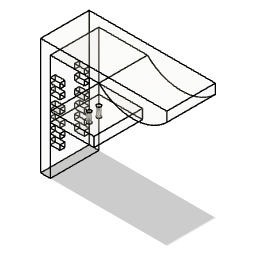
clamp v5 (Autodesk Fusion 360 design; units mm, degrees)
Autodesk Fusion 360 part; units mm, degrees
sketch "草图1" plane through (0, 0, 0) normal (0, 1, 0) x (1, 0, 0) in component "Component"
  line L0 (-30, 25) -> (30, 25)
  line L1 (30, 25) -> (30, -25)
  line L2 (30, -25) -> (-30, -25)
  line L3 (-30, -25) -> (-30, 25)
  line L4 (-30, 25) -> (30, -25) construction
  line L5 (30, 25) -> (-30, -25) construction
  dimension "d1" = 60
  dimension "d2" = 50
  constraint horizontal L0
  constraint perpendicular L0 L1
  constraint parallel L0 L2
  constraint parallel L1 L3
  constraint coincident L4 origin
  constraint coincident L5 origin
  measures "d1" distance of L0.start L0.end
  measures "d2" distance of L0.start L2.end
extrude "拉伸1" add sketch "草图1" along normal blind 10 makes body 1 in component "Component"
sketch "草图2" plane through (0, 10, 0) normal (0, 1, 0) x (-1, 0, 0) in component "Component"
  line L0 (30, 25) -> (-30, 25)
  line L1 (-30, 25) -> (-30, -25)
  line L2 (-30, -25) -> (30, -25)
  line L3 (30, -25) -> (30, 25)
  line L4 (30, -25) -> (20, -25)
  line L5 (20, -25) -> (20, 25)
  line L6 (20, 25) -> (30, 25)
  line L7 (30, 25) -> (30, -25)
  dimension "d5" = 10
  constraint horizontal L4
  constraint vertical L5
  constraint horizontal L6
  constraint vertical L7
  constraint coincident L0 L5.end
  constraint coincident L2.end L3.start
  measures "d5" distance of L2.end L4.end
extrude "拉伸2" add sketch "草图2" along normal blind 60 contours L0 L2 L3 L4 L5 L6 L7 bodies 1 in component "Component"
sketch "草图3" plane through (-20, 0, 0) normal (1, 0, 0) x (0, 0, -1) in component "Component"
  line L0 (-25, 10) -> (25, 10)
  line L1 (25, 10) -> (25, 70)
  line L2 (25, 70) -> (-25, 70)
  line L3 (-25, 70) -> (-25, 10)
  line L4 (-25, 70) -> (25, 70)
  line L5 (25, 70) -> (25, 60)
  line L6 (25, 60) -> (-25, 60)
  line L7 (-25, 60) -> (-25, 70)
  dimension "d8" = 10
  constraint horizontal L4
  constraint vertical L5
  constraint horizontal L6
  constraint vertical L7
  constraint coincident L1 L5.end
  constraint coincident L2.end L3.start
  measures "d8" distance of L2.end L6.end
extrude "拉伸3" add sketch "草图3" along normal blind 120 contours L1 L2 L3 L4 L5 L6 L7 bodies 1 in component "Component"
sketch "草图1 (2)" plane through (0, 0, 25) normal (0, 0, 1) x (1, 0, 0)
  line L0 (-30, 0) -> (30, 0)
  line L1 (30, 0) -> (30, 10)
  line L2 (30, 10) -> (-20, 10)
  line L3 (-20, 10) -> (-20, 60)
  line L4 (-20, 60) -> (100, 60)
  line L5 (100, 60) -> (100, 70)
  line L6 (100, 70) -> (-30, 70)
  line L7 (-30, 70) -> (-30, 0)
  arc A0 (30, 60) -> (100, 60) centre (65, 95.7071) ccw
  dimension "d14" = 50
  dimension "d15" = 50
  constraint coincident L4.end L5.start
  constraint coincident L4 A0.start
  measures "d14" radius of A0
  measures "d15" distance of L3.end A0.start
extrude "拉伸4" add sketch "草图1 (2)" against normal blind 50 contours L4 A0 bodies 1 in component "Component"
sketch "草图2 (2)" plane through (0, 0, 0) normal (0, -1, 0) x (1, 0, 0)
  line L0 (30, 25) -> (-30, 25)
  line L1 (-30, 25) -> (-30, -25)
  line L2 (-30, -25) -> (30, -25)
  line L3 (30, -25) -> (30, 25)
  line L4 (-20, -25) -> (-20, 25)
  line L5 (-30, 25) -> (-20, 25)
  line L6 (-20, 25) -> (-20, -25)
  line L7 (-20, -25) -> (-30, -25)
  line L8 (-30, -25) -> (-30, 25)
  constraint horizontal L5
  constraint vertical L6
  constraint horizontal L7
  constraint vertical L8
  constraint coincident L4.start L6.end
  constraint coincident L0.end L1.start
extrude "拉伸5" add sketch "草图2 (2)" along normal blind 50 contours L0 L1 L2 L4 L5 L6 L7 L8 bodies 1 in component "Component"
sketch "草图3 (2)" plane through (0, 0, 0) normal (0, -1, 0) x (1, 0, 0)
  line L0 (-20, 25) -> (-20, -25)
  line L1 (-20, -25) -> (30, -25)
  line L2 (30, -25) -> (30, 25)
  line L3 (30, 25) -> (-20, 25)
  dimension "d21" = 20
  measures "d21" distance of origin L0
ref_plane "工作平面2" through (-20, 0, 0) normal (1, 0, 0) x (0, 1, 0)
split "分割1" by plane through (-20, 0, 0) normal (1, 0, 0) bodies 1 makes body 2 at (20, 70, -8.3333) makes body 3 at (-3.3333, 0, -8.3333) in component "Component"
combine "合并1" operation add target body 2 tool bodies 1 in component "Component"
sketch "草图4" plane through (-20, 0, 0) normal (-1, 0, 0) x (0, 0, 1)
  line L0 (25, 10) -> (-25, 10)
  line L1 (-25, 10) -> (-25, 0)
  line L2 (-25, 0) -> (25, 0)
  line L3 (25, 0) -> (25, 10)
  line L4 (-15, 7) -> (-10, 7)
  line L5 (-10, 7) -> (-10, 2)
  line L6 (-10, 2) -> (-15, 2)
  line L7 (-15, 2) -> (-15, 7)
  line L8 (10, 7) -> (15, 7)
  line L9 (15, 7) -> (15, 2)
  line L10 (15, 2) -> (10, 2)
  line L11 (10, 2) -> (10, 7)
  dimension "d24" = 5
  dimension "d25" = 5
  dimension "d26" = 5
  dimension "d27" = 10
  dimension "d28" = 3
  dimension "d29" = 5
  dimension "d30" = 5
  dimension "d31" = 10
  dimension "d32" = 3
  constraint horizontal L4
  constraint vertical L5
  constraint horizontal L6
  constraint vertical L7
  constraint horizontal L8
  constraint vertical L9
  constraint horizontal L10
  constraint vertical L11
  measures "d24" distance of L4.start L4.end
  measures "d25" distance of L4.start L6.end
  measures "d26" distance of L4.start L4.end
  measures "d27" distance of origin L5
  measures "d28" distance of L0 L4
  measures "d29" distance of L8.start L8.end
  measures "d30" distance of L8.start L10.end
  measures "d31" distance of L11 origin
  measures "d32" distance of L0 L8
extrude "拉伸6" add sketch "草图4" along normal blind 8 contours L4 L5 L6 L7 | L8 L9 L10 L11 bodies 3 in component "Component"
sketch "草图5" plane through (-20, 0, 0) normal (1, 0, 0) x (0, 0, -1)
  line L0 (25, 60) -> (-25, 60)
  line L1 (-25, 60) -> (-25, -50)
  line L2 (-25, -50) -> (25, -50)
  line L3 (25, -50) -> (25, 60)
  line L4 (-10, 2) -> (-15, 2)
  line L5 (-15, 2) -> (-15, 7)
  line L6 (-15, 7) -> (-10, 7)
  line L7 (-10, 7) -> (-10, 2)
  line L8 (15, 2) -> (10, 2)
  line L9 (10, 2) -> (10, 7)
  line L10 (10, 7) -> (15, 7)
  line L11 (15, 7) -> (15, 2)
  line L12 (-15, 7) -> (-10, 7)
  line L13 (-10, 7) -> (-10, 2)
  line L14 (-10, 2) -> (-15, 2)
  line L15 (-15, 2) -> (-15, 7)
  line L16 (10, 7) -> (15, 7)
  line L17 (15, 7) -> (15, 2)
  line L18 (15, 2) -> (10, 2)
  line L19 (10, 2) -> (10, 7)
  constraint horizontal L12
  constraint vertical L13
  constraint horizontal L14
  constraint vertical L15
  constraint coincident L4.start L7.end
  constraint coincident L5.end L6.start
  constraint horizontal L16
  constraint vertical L17
  constraint horizontal L18
  constraint vertical L19
  constraint coincident L8.start L11.end
  constraint coincident L9.end L10.start
extrude "拉伸7" cut sketch "草图5" against normal blind 10 contours L4 L5 L6 L7 L12 L13 L14 L15 | L8 L9 L10 L11 L16 L17 L18 L19 bodies 2 in component "Component"
extrude "拉伸8" add 2 faces at (-28, 5.3333, 11.6667) (-28, 5.3333, -13.3333) along direction (-1, 0, 0) blind 2 on bodies 3 bodies 3 in component "Component"
sketch "草图6" plane through (-30, 0, 0) normal (-1, 0, 0) x (0, 0, 1)
  line L0 (10, 2) -> (10, 7)
  line L1 (10, 7) -> (15, 7)
  line L2 (15, 7) -> (15, 2)
  line L3 (15, 2) -> (10, 2)
  line L4 (-15, 2) -> (-15, 7)
  line L5 (-15, 7) -> (-10, 7)
  line L6 (-10, 7) -> (-10, 2)
  line L7 (-10, 2) -> (-15, 2)
  line L8 (25, -50) -> (25, 70)
  line L9 (25, 70) -> (-25, 70)
  line L10 (-25, 70) -> (-25, -50)
  line L11 (-25, -50) -> (25, -50)
  line L12 (-15, 20) -> (-10, 20)
  line L13 (-10, 20) -> (-10, 15)
  line L14 (-10, 15) -> (-15, 15)
  line L15 (-15, 15) -> (-15, 20)
  line L16 (10, 20) -> (15, 20)
  line L17 (15, 20) -> (15, 15)
  line L18 (15, 15) -> (10, 15)
  line L19 (10, 15) -> (10, 20)
  line L20 (-15, 30) -> (-10, 30)
  line L21 (-10, 30) -> (-10, 25)
  line L22 (-10, 25) -> (-15, 25)
  line L23 (-15, 25) -> (-15, 30)
  line L24 (10, 30) -> (15, 30)
  line L25 (15, 30) -> (15, 25)
  line L26 (15, 25) -> (10, 25)
  line L27 (10, 25) -> (10, 30)
  line L28 (-15, -5) -> (-10, -5)
  line L29 (-10, -5) -> (-10, -10)
  line L30 (-10, -10) -> (-15, -10)
  line L31 (-15, -10) -> (-15, -5)
  line L32 (10, -5) -> (15, -5)
  line L33 (15, -5) -> (15, -10)
  line L34 (15, -10) -> (10, -10)
  line L35 (10, -10) -> (10, -5)
  line L36 (-15, -15) -> (-10, -15)
  line L37 (-10, -15) -> (-10, -20)
  line L38 (-10, -20) -> (-15, -20)
  line L39 (-15, -20) -> (-15, -15)
  line L40 (10, -15) -> (15, -15)
  line L41 (15, -15) -> (15, -20)
  line L42 (15, -20) -> (10, -20)
  line L43 (10, -20) -> (10, -15)
  line L44 (-15, -25) -> (-10, -25)
  line L45 (-10, -25) -> (-10, -30)
  line L46 (-10, -30) -> (-15, -30)
  line L47 (-15, -30) -> (-15, -25)
  line L48 (10, -25) -> (15, -25)
  line L49 (15, -25) -> (15, -30)
  line L50 (15, -30) -> (10, -30)
  line L51 (10, -30) -> (10, -25)
  dimension "d39" = 5
  dimension "d40" = 5
  dimension "d41" = 5
  dimension "d42" = 5
  dimension "d43" = 5
  dimension "d44" = 5
  dimension "d45" = 5
  dimension "d46" = 5
  dimension "d47" = 5
  dimension "d48" = 5
  dimension "d49" = 5
  dimension "d50" = 5
  dimension "d51" = 5
  dimension "d52" = 5
  dimension "d53" = 5
  dimension "d54" = 5
  dimension "d55" = 5
  dimension "d56" = 5
  dimension "d57" = 15
  dimension "d58" = 10
  dimension "d59" = 20
  dimension "d60" = 5
  dimension "d61" = 5
  dimension "d62" = 30
  dimension "d64" = 15
  constraint horizontal L12
  constraint vertical L13
  constraint horizontal L14
  constraint vertical L15
  constraint horizontal L16
  constraint vertical L17
  constraint horizontal L18
  constraint vertical L19
  constraint horizontal L20
  constraint vertical L21
  constraint horizontal L22
  constraint vertical L23
  constraint horizontal L24
  constraint vertical L25
  constraint horizontal L26
  constraint vertical L27
  constraint horizontal L28
  constraint vertical L29
  constraint horizontal L30
  constraint vertical L31
  constraint horizontal L32
  constraint vertical L33
  constraint horizontal L34
  constraint vertical L35
  constraint horizontal L36
  constraint vertical L37
  constraint horizontal L38
  constraint vertical L39
  constraint horizontal L40
  constraint vertical L41
  constraint horizontal L42
  constraint vertical L43
  constraint horizontal L44
  constraint vertical L45
  constraint horizontal L46
  constraint vertical L47
  constraint horizontal L48
  constraint vertical L49
  constraint horizontal L50
  constraint vertical L51
  constraint vertical L6.end L21.end
  constraint vertical L6.end L13.end
  constraint vertical L0.end L18.end
  constraint vertical L0.end L26.end
  constraint horizontal L13.end L18.end
  constraint horizontal L21.end L26.end
  constraint vertical L0.start L32.start
  constraint vertical L32.start L40.start
  constraint vertical L42.end L48.start
  constraint vertical L6.end L28.end
  constraint vertical L29.end L36.end
  constraint vertical L37.end L44.end
  constraint horizontal L28.end L32.start
  constraint horizontal L36.end L40.start
  constraint horizontal L44.end L48.start
  measures "d39" distance of L20.start L20.end
  measures "d40" distance of L20.start L22.end
  measures "d41" distance of L24.start L24.end
  measures "d42" distance of L24.end L25.end
  measures "d43" distance of L16.start L16.end
  measures "d44" distance of L16.start L18.end
  measures "d45" distance of L32.start L32.end
  measures "d46" distance of L32.start L34.end
  measures "d47" distance of L28.start L28.end
  measures "d48" distance of L28.start L30.end
  measures "d49" distance of L36.start L36.end
  measures "d50" distance of L36.start L38.end
  measures "d51" distance of L44.start L44.end
  measures "d52" distance of L44.end L45.end
  measures "d53" distance of L48.start L48.end
  measures "d54" distance of L48.start L50.end
  measures "d55" distance of L40.start L40.end
  measures "d56" distance of L40.start L42.end
  measures "d57" distance of origin L14
  measures "d58" distance of L10 L15
  measures "d59" distance of origin L12
  measures "d60" distance of L12 L22
  measures "d61" distance of origin L28
  measures "d62" distance of origin L46
  measures "d64" distance of origin L36
extrude "拉伸9" cut sketch "草图6" against normal blind 10 contours L12 L13 L14 L15 | L16 L17 L18 L19 | L20 L21 L22 L23 | L24 L25 L26 L27 | L28 L29 L30 L31 | L32 L33 L34 L35 | L36 L37 L38 L39 | L40 L41 L42 L43 | L44 L45 L46 L47 | L48 L49 L50 L51 bodies 2 in component "Component"
sketch "草图7" plane through (0, 0, 0) normal (0, -1, 0) x (1, 0, 0)
  circle A0 centre (0, -5) radius 2.5
  circle A1 centre (0, 5) radius 2.5
  line L0 (1.75, 0) -> (22.5, 0)
  dimension "d67" = 5
  dimension "d68" = 5
  dimension "d69" = 10
  constraint symmetric A0 A1 L0
  measures "d67" diameter of A0
  measures "d68" diameter of A1
  measures "d69" distance of A0.centre A1.centre
extrude "拉伸10" cut sketch "草图7" against normal blind 10 bodies 3 in component "Component"
thread "螺纹2" "ISO Metric profile 5.0 M5x0.8 6H" major diameter 5.12 minor diameter 4.234 pitch 0.8 angle 60 resizes the face on face at (2.4969, 6.6667, -5.1246) on bodies 3 in component "Component"
thread "螺纹3" "ISO Metric profile 5.0 M5x0.8 6H" major diameter 5.12 minor diameter 4.234 pitch 0.8 angle 60 resizes the face on face at (2.4969, 6.6667, 4.8754) on bodies 3 in component "Component"
sketch "草图4 (2)" plane through (0, 0, 0) normal (0, -1, 0) x (1, 0, 0) in component "Component"
  line L0 (25, 25) -> (25, -25)
  line L1 (25, 25) -> (30, 25)
  line L2 (30, 25) -> (30, -25)
  line L3 (30, -25) -> (25, -25)
  point P0 (30, -25)
  dimension "d72" = 5
  dimension "d73" = 50
  constraint vertical L0
  constraint perpendicular L0 L1
  constraint coincident P0 L2.end
  constraint perpendicular L1 L2
  constraint perpendicular L0 L3
  measures "d72" distance of L0.end P0
  measures "d73" distance of L0.start L0.end
extrude "拉伸11" cut sketch "草图4 (2)" against normal blind 10 bodies 3 in component "Component"
component "Component" placed x (1, 0, 0) y (0, 1, 0) z (0, 0, 1) at (0, 0, 0)
